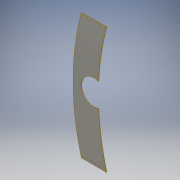
# Autodesk Inventor part: Floor
Saved by Autodesk Inventor 2016 (Build 200138000, 138)
## iProperties
Created: 2016-04-15
Part Number: Floor
Material: Generic
Document SubType Name: Modeling
Designer: 3DPrinterUser
Density: 1 g/cm^3
Appearance: Titanium
Author: 3DPrinterUser
Autodesk Inventor part; units mm, degrees
ref_plane "YZ Plane" through (0, 0, 0) normal (1, 0, 0) x (0, 1, 0)
ref_plane "XZ Plane" through (0, 0, 0) normal (0, 1, 0) x (-1, 0, 0)
ref_plane "XY Plane" through (0, 0, 0) normal (0, 0, 1) x (1, 0, 0)
sketch "Sketch1" plane through (0, 0, 0) normal (0, 1, 0) x (-1, 0, 0)
  arc A0 (0, -750) -> (0, 750) centre (-2762.5, 0) ccw construction
  line L0 (-22.4292, 0) -> (36.1533, 0) construction
  line L1 (0, 750) -> (0, -750) construction
  line L2 (150, 750) -> (-150, 750)
  line L3 (150, -750) -> (-150, -750)
  arc A1 (150, -750) -> (150, 750) centre (-2612.5, 0) ccw
  arc A2 (-150, -750) -> (-150, 750) centre (-2912.5, 0) ccw
  point P0 (0, 0)
  point P1 (100, 0)
  point P2 (250, 0)
  point P3 (-50, 0)
  dimension "d0" = 1500
  dimension "d1" = 100
  dimension "d2" = 300
  dimension "d3" = 150
  dimension "d4" = 150
  constraints: 9 point on circle, 8 end point, 4 symmetric about line, 3 centre point, 2 horizontal, 2 midpoint, 2 point on line, 1 vertical
  measures "d0" distance of L1.start L1.end
  measures "d1" distance of point (0, 0) point (100, 0)
  measures "d2" distance of L2.start L2.end
  measures "d3" distance of point (100, 0) point (250, 0)
  measures "d4" distance of point (100, 0) point (-50, 0)
extrude "Extrusion1" add sketch "Sketch1" along normal blind 5
sketch "Sketch2" plane through (0, 5, 0) normal (0, 1, 0) x (1, 0, 0)
  line L0 (-150, -750) -> (150, -750) construction
  arc A0 (150, 750) -> (150, -750) centre (2912.5, 0) ccw construction
  line L1 (150, 750) -> (-150, 750) construction
  arc A1 (-150, 750) -> (-150, -750) centre (2612.5, 0) ccw construction
  line L2 (-150, -750) -> (150, -750) construction
  arc A2 (150, 750) -> (150, -750) centre (2912.5, 0) ccw construction
  line L3 (150, -750) -> (150, -750) construction
  line L4 (150, -750) -> (150, -750) construction
  line L5 (150, 750) -> (-150, 750) construction
  line L6 (150, -750) -> (150, 750) construction
  circle A3 centre (0, 0) radius 150
  line L7 (150, 0) -> (-250, 0) construction
  arc A4 (-150, 750) -> (-150, -750) centre (2612.5, 0) ccw construction
  circle A5 centre (0, 0) radius 36 construction
  point P0 (-36, 0)
  point P1 (-18, -31.1769)
  point P2 (18, -31.1769)
  point P3 (36, 0)
  point P4 (18, 31.1769)
  point P5 (-18, 31.1769)
  dimension "d42" = 72
  dimension "d9" = 300
  dimension "d45" = 360
  constraints: 8 end point, 2 point on circle, 2 point on line, 2 vertical, 1 centre point, 1 horizontal alignment, 1 midpoint, 1 perpendicular, 1 tangent, 9 other
  measures "d9" diameter of A3
extrude "Extrusion2" cut sketch "Sketch2" against normal through all
sketch "Sketch3" plane through (0, 5, 0) normal (0, 1, 0) x (1, 0, 0)
  line L0 (-150, -750) -> (150, -750) projected
  arc A0 (53.4335, -140.1601) -> (150, -750) centre (2912.5, 0) ccw projected
  line L1 (150, 750) -> (-150, 750) projected
  arc A1 (-150, 750) -> (-150, -750) centre (2612.5, 0) ccw projected
  line L2 (-137.7375, -734) -> (129.1556, -734)
  arc A2 (129.1556, 734) -> (129.1556, -734) centre (2912.5, 0) ccw
  line L3 (129.1556, 734) -> (-137.7375, 734)
  arc A3 (-137.7375, 734) -> (-137.7375, -734) centre (2612.5, 0) ccw
  line L4 (-141.9579, -718) -> (124.9853, -718)
  arc A4 (53.4335, 140.1601) -> (53.4335, -140.1601) centre (0, 0) ccw projected
  arc A5 (150, 750) -> (53.4335, 140.1601) centre (2912.5, 0) ccw projected
  point P0 (0, 0)
  point P1 (-84.3589, -734)
  point P2 (-30.9803, -734)
  point P3 (22.3983, -734)
  point P4 (75.777, -734)
  point P5 (129.1556, -734)
  point P6 (-88.5793, -718)
  point P7 (-35.2007, -718)
  point P8 (18.1779, -718)
  point P9 (71.5566, -718)
  point P10 (124.9352, -718)
  dimension "d10" = 16
  dimension "d11" = 266.8931
  dimension "d14" = 53.3786
  dimension "d26" = 16
  dimension "d27" = 16
  dimension "d30" = 53.3786
  constraints: 6 end point, 6 point on circle, 3 horizontal, 2 centre point, 2 coincident, 13 other
  measures "d10" radial gap between concentric circles of A1 A3
  measures "d11" distance of L2.start L2.end
  measures "d14" distance of point (-137.737, -734) point (-84.359, -734)
  measures "d26" distance between parallel lines of L2 L0
  measures "d27" distance between parallel lines of L4 L2
  measures "d30" distance of point (-141.958, -718) point (-88.579, -718)
hole "Hole2" at (-137.7375, 5, 734) at (-84.3589, 5, 734) at (-30.9803, 5, 734) at (22.3983, 5, 734) at (75.777, 5, 734) at (129.1556, 5, 734) at (-141.9579, 5, 718) at (-88.5793, 5, 718) at (-35.2007, 5, 718) at (18.1779, 5, 718) at (71.5566, 5, 718) at (124.9352, 5, 718) direction (0, -1, 0) diameter 6.2 end through all
mirror "Mirror1" about plane through (0, 0, 0) normal (0, 0, 1) of "Hole2"
equation "\"d3\" = 0.5 * d2"
equation "\"d4\" = 0.5 * d2"
equation "\"d14\" = 0.2 * d11"
equation "\"d27\" = d26"
equation "\"d30\" = 0.2 * d11"
body "Solid1"
